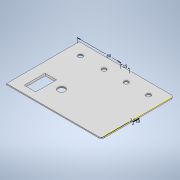
# Autodesk Inventor part: Fascia
Saved by Autodesk Inventor 2021 (Build 250183000, 183)
## iProperties
Created: 2021-02-27
Part Number: Fascia
Material: Generisch
Document SubType Name: Modeling
Designer: michox
Density: 1 g/cm^3
Appearance: Vorgabe
Author: michox
Autodesk Inventor part; units mm, degrees
ref_plane "YZ Plane" through (0, 0, 0) normal (1, 0, 0) x (0, 1, 0)
ref_plane "XZ Plane" through (0, 0, 0) normal (0, 1, 0) x (-1, 0, 0)
ref_plane "XY Plane" through (0, 0, 0) normal (0, 0, 1) x (1, 0, 0)
sketch "Skizze1" plane through (0, 0, 0) normal (0, 1, 0) x (-1, 0, 0)
  line L0 (0, 0) -> (150, 0)
  line L1 (150, 0) -> (150, -120)
  line L2 (150, -120) -> (0, -120)
  line L3 (0, -120) -> (0, 0)
  circle A0 centre (137, -98.5) radius 4
  circle A1 centre (94, -98.5) radius 4
  circle A2 centre (53.5, -98.5) radius 4
  circle A3 centre (13, -98.5) radius 4
  line L4 (140, -3) -> (123, -3)
  line L5 (123, -3) -> (123, -37)
  line L6 (123, -37) -> (140, -37)
  line L7 (140, -37) -> (140, -3)
  circle A4 centre (101.5, -28.5) radius 6.5
  dimension "d0" = 150
  dimension "d1" = 120
  dimension "d2" = 8
  dimension "d3" = 98.5
  dimension "d4" = 13
  dimension "d5" = 8
  dimension "d6" = 8
  dimension "d7" = 8
  dimension "d8" = 56
  dimension "d9" = 96.5
  dimension "d10" = 137
  dimension "d11" = 17
  dimension "d12" = 34
  dimension "d13" = 3
  dimension "d14" = 10
  dimension "d15" = 13
  dimension "d16" = 28.5
  dimension "d17" = 48.5
  constraints: 16 end point, 5 centre point, 4 parallel, 2 horizontal, 2 perpendicular
  measures "d0" distance of L1.end L2.end
  measures "d1" distance of L2.end L0.start
  measures "d2" diameter of A0
  measures "d3" distance from line of A0.centre L0
  measures "d4" distance from line of L1 A0.centre
  measures "d5" diameter of A1
  measures "d6" diameter of A2
  measures "d7" diameter of A3
  measures "d8" distance from line of A1.centre L1
  measures "d9" distance from line of A2.centre L1
  measures "d10" distance from line of A3.centre L1
  measures "d11" distance of L6.end L5.end
  measures "d12" distance of L5.end L4.end
  measures "d13" distance between parallel lines of L4 L0
  measures "d14" distance between parallel lines of L1 L7
  measures "d15" diameter of A4
  measures "d16" distance from line of L0 A4.centre
  measures "d17" distance from line of L1 A4.centre
extrude "Extrusion1" add sketch "Skizze1" along normal blind 2
chamfer "Fase1" distance 2 angle 45 4 edges at (-140, 2, -20) (-131.5, 2, -37) (-123, 2, -20) (-131.5, 2, -3)
sketch "Skizze2" plane through (0, 0, 0) normal (0, -1, 0) x (1, 0, 0)
  circle A0 centre (-101.8979, -9.7616) radius 3.5
  circle A1 centre (-3.5, -87) radius 3.5
  circle A2 centre (-3.5, -3.5) radius 3.5
  line L0 (0, 0) -> (0, -120) projected
  line L1 (0, -120) -> (-150, -120) projected
  line L2 (-150, 0) -> (0, 0) projected
  circle A3 centre (-146.5, -87) radius 3.5
  line L3 (-150, -120) -> (-150, 0) projected
  dimension "d23" = 7
  dimension "d24" = 7
  dimension "d25" = 7
  dimension "d26" = 3.5
  dimension "d28" = 3.5
  dimension "d29" = 3.5
  dimension "d30" = 7
  dimension "d31" = 3.5
  dimension "d32" = 87
  dimension "d33" = 87
  constraints: 4 centre point
  measures "d23" diameter of A0
  measures "d24" diameter of A1
  measures "d25" diameter of A2
  measures "d26" distance from line of L0 A1.centre
  measures "d28" distance from line of L2 A2.centre
  measures "d29" distance from line of L0 A2.centre
  measures "d30" diameter of A3
  measures "d31" distance from line of L3 A3.centre
  measures "d32" distance from line of A1.centre L2
  measures "d33" distance from line of A3.centre L2
extrude "Extrusion2" add sketch "Skizze2" along normal blind 4.5 contours A0 | A1 | A3 | A2
sketch "Skizze3" plane through (-101.8979, -4.5, -9.7616) normal (0, -1, 0) x (1, 0, 0)
  circle A0 centre (0, 0) radius 3.5 projected
  circle A1 centre (98.3979, 6.2616) radius 3.5 projected
  point P0 (101.8979, 9.7616)
extrude "Extrusion3" add sketch "Skizze3" along normal blind 2.5
sketch "Skizze4" plane through (-146.5, -4.5, -87) normal (0, -1, 0) x (1, 0, 0)
  circle A0 centre (143, 0) radius 3.5 projected
  point P0 (146.5, 87)
  constraints: 1 coincident
hole "Bohrung1" at (-3.5, -4.5, -87) direction (0, 1, 0) diameter 3 depth 5
sketch "Skizze5" plane through (-3.5, -7, -3.5) normal (0, -1, 0) x (1, 0, 0)
  circle A0 centre (0, 0) radius 3.5 projected
  point P0 (3.5, 3.5)
  constraints: 1 coincident
hole "Bohrung2" at (-3.5, -7, -3.5) direction (0, 1, 0) diameter 3 depth 7
sketch "Skizze6" plane through (-101.8979, -7, -9.7616) normal (0, -1, 0) x (1, 0, 0)
  circle A0 centre (0, 0) radius 3.5 projected
  point P0 (101.8979, 9.7616)
  constraints: 1 coincident
hole "Bohrung3" at (-101.8979, -7, -9.7616) direction (0, 1, 0) diameter 3 depth 7
sketch "Skizze7" plane through (-146.5, -4.5, -87) normal (0, -1, 0) x (1, 0, 0)
  circle A0 centre (0, 0) radius 3.5 projected
  point P0 (146.5, 87)
  constraints: 1 coincident
hole "Bohrung4" at (-146.5, -4.5, -87) direction (0, 1, 0) diameter 3 depth 5
sketch "Skizze8" plane through (0, 0, 0) normal (0, -1, 0) x (1, 0, 0)
  line L0 (0, -120) -> (-150, -120) projected
  line L1 (0, -120) -> (12, -120)
  line L2 (12, -120) -> (12, 0)
  line L3 (12, 0) -> (0, 0)
  line L4 (0, 0) -> (0, -120)
  circle A0 centre (-13, -98.5) radius 4 projected
  circle A1 centre (-137, -98.5) radius 4 projected
  line L5 (-150, 0) -> (-162, 0)
  line L6 (-162, 0) -> (-162, -120)
  line L7 (-162, -120) -> (-150, -120)
  line L8 (-150, -120) -> (-150, 0)
  line L9 (-150, -120) -> (-150, -87) projected
  line L10 (-162, 0) -> (12, 0)
  line L11 (12, 0) -> (12, 12.2394)
  line L12 (12, 12.2394) -> (-162, 12.2394)
  line L13 (-162, 12.2394) -> (-162, 0)
  point P0 (0, 0)
  point P1 (0, 0)
  dimension "d66" = 25
  dimension "d67" = 25
  constraints: 24 end point, 6 parallel, 3 horizontal, 3 perpendicular, 1 collinear
  measures "d66" distance from line of L2 A0.centre
  measures "d67" distance from line of A1.centre L6
extrude "Extrusion4" add sketch "Skizze8" against normal blind 2 contours L4 L3 L2 L1 | L7 L6 L5 L8 | L10 L5 L13 L12 L11 L3
sketch "Skizze9" plane through (0, 0, 0) normal (0, -1, 0) x (1, 0, 0)
  circle A0 centre (-3.5, -3.5) radius 3.5 projected
  circle A1 centre (-3.5, -87) radius 3.5 projected
  circle A2 centre (-101.8979, -9.7616) radius 3.5 projected
  circle A3 centre (-137, -98.5) radius 4 projected
  circle A4 centre (-94, -98.5) radius 4 projected
  circle A5 centre (-53.5, -98.5) radius 4 projected
  circle A6 centre (-13, -98.5) radius 4 projected
  circle A7 centre (-101.5, -28.5) radius 6.5 projected
  line L0 (-140, -3) -> (-140, -37) projected
  line L1 (-123, -3) -> (-140, -3) projected
  line L2 (-123, -37) -> (-123, -3) projected
  line L3 (-140, -37) -> (-123, -37) projected
  circle A8 centre (-146.5, -87) radius 3.5 projected
  line L4 (9.3, -117.3) -> (-162, -117.3)
  line L5 (9.3, -117.3) -> (9.3, 9.5394)
  line L6 (9.3, 9.5394) -> (-162, 9.5394)
  line L7 (-162, 9.5394) -> (-162, -117.3)
  line L8 (12, -120) -> (12, 12.2394) projected
  line L9 (12, 12.2394) -> (-162, 12.2394) projected
  line L10 (-162, 12.2394) -> (-162, -120) projected
  line L11 (12, -120) -> (-162, -120) projected
  line L12 (-160, 7.5394) -> (7.3, 7.5394)
  line L13 (7.3, 7.5394) -> (7.3, -115.3)
  line L14 (7.3, -115.3) -> (-160, -115.3)
  line L15 (-160, -115.3) -> (-160, 7.5394)
  line L16 (-160, -115.3) -> (-160, -117.3)
  point P0 (0, 0)
  dimension "d70" = 2.7
  dimension "d71" = 2.7
  dimension "d72" = 0
  dimension "d73" = 2.7
  dimension "d74" = 2
  dimension "d75" = 2
  dimension "d76" = 2
  dimension "d77" = 2
  dimension "d81" = 132.2394
  constraints: 18 end point, 9 centre point, 2 parallel, 2 perpendicular, 1 horizontal, 1 point on line
  measures "d70" distance between parallel lines of L8 L5
  measures "d71" distance between parallel lines of L6 L9
  measures "d72" distance between parallel lines of L10 L7
  measures "d73" distance between parallel lines of L11 L4
  measures "d74" distance between parallel lines of L5 L13
  measures "d75" distance between parallel lines of L6 L12
  measures "d76" distance between parallel lines of L7 L15
  measures "d77" distance between parallel lines of L4 L14
  measures "d81" distance between parallel lines of L11 L9
extrude "Extrusion5" add sketch "Skizze9" along normal blind 2 contours L4 L7 L6 L5
fillet "Rundung1" radius 4.75 4 edges at (12, 1, -120) (9.3, -1, -117.3) (12, 1, 12.2394) (9.3, -1, 9.5394)
sketch "Skizze10" plane through (9.3, 0, 4.7894) normal (1, 0, 0) x (0, 0, -1)
  line L0 (122.0894, 0) -> (-4.75, 0) projected
  line L1 (53.6697, 0) -> (63.6697, 0)
  line L2 (63.6697, 0) -> (63.6697, -3.5)
  line L3 (63.6697, -3.5) -> (53.6697, -3.5)
  line L4 (53.6697, -3.5) -> (53.6697, 0)
  line L5 (58.6697, -3.5) -> (58.6697, 0)
  line L6 (-2.7, 2) -> (120.0394, 2) projected
  line L7 (0, 0) -> (117.3394, 0) projected
  line L8 (53.6697, -2.5) -> (63.6697, -2.5)
  point P0 (4.7894, 0)
  dimension "d83" = 1
  dimension "d91" = 10
  dimension "d92" = 2.5
  constraints: 12 end point, 3 point on line, 2 midpoint, 2 parallel, 2 perpendicular, 1 horizontal
  measures "d83" distance between parallel lines of L8 L3
  measures "d91" distance of L2.end L3.end
  measures "d92" distance between parallel lines of L0 L8
extrude "Extrusion6" add sketch "Skizze10" against normal blind 2
extrude "Extrusion7" add sketch "Skizze10" along normal blind 0.4 contours L2 L3 L5 L8 | L5 L3 L4 L8
chamfer "Fase2" distance 0.25 angle 45 2 edges at (9.7, -2.5, -53.8803) (9.7, -3.5, -53.8803)
chamfer "Fase3" distance 2 angle 30 1 edges at (-162, 2, -53.8803) measured on face at (-162, 1.5, -53.8803)
sketch "Skizze11" plane through (9.3, 0, 4.7894) normal (1, 0, 0) x (0, 0, -1)
  line L0 (117.3394, 0) -> (117.3394, -2) projected
  line L1 (117.3394, 0) -> (105.2695, 0)
  line L2 (105.2695, 0) -> (105.2695, -2)
  line L3 (105.2695, -2) -> (117.3394, -2)
  line L4 (117.3394, -2) -> (117.3394, 0)
  point P0 (4.7894, 0)
  constraints: 8 end point, 2 parallel, 1 horizontal, 1 perpendicular
extrude "Extrusion8" cut sketch "Skizze11" against normal blind 3.2
sketch "Skizze12" plane through (4.55, -2, -117.3) normal (0, 0, -1) x (-1, 0, 0)
  line L0 (164.55, 0) -> (-2.75, 0) projected
  line L1 (0, 2) -> (166.55, 2) projected
  line L2 (86.55, 0) -> (71.55, 0)
  line L3 (71.55, 0) -> (71.55, 2)
  line L4 (71.55, 2) -> (86.55, 2)
  line L5 (86.55, 2) -> (86.55, 0)
  line L6 (166.55, 2) -> (166.55, 0) projected
  point P0 (4.55, 2)
  dimension "d98" = 15
  dimension "d99" = 80
  constraints: 8 end point, 2 parallel, 2 point on line, 1 horizontal, 1 perpendicular
  measures "d98" distance of L3.end L4.end
  measures "d99" distance between parallel lines of L5 L6
